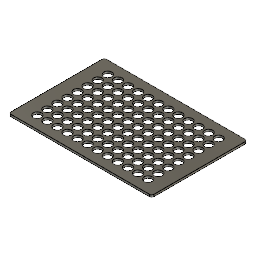
PlateAdaptor_gasket (Autodesk Fusion 360 design; units mm, degrees)
Autodesk Fusion 360 part; units mm, degrees
sketch "Sketch1" plane through (0, 0, 0) normal (0, 0, 1) x (1, 0, 0)
  line L0 (-61.88, 42.735) -> (61.88, 42.735)
  line L1 (63.88, 40.735) -> (63.88, -40.735)
  line L2 (61.88, -42.735) -> (-61.88, -42.735)
  line L3 (-63.88, -40.735) -> (-63.88, 40.735)
  line L4 (-63.88, 42.735) -> (63.88, -42.735) construction
  line L5 (63.88, 42.735) -> (-63.88, -42.735) construction
  line L6 (-48.38, 42.735) -> (-58.38, 42.735)
  line L7 (48.38, -47.37) -> (58.38, -47.37)
  line L8 (-58.38, -47.37) -> (-48.38, -47.37)
  line L9 (-49.5, 31.5) -> (49.5, 31.5)
  line L10 (49.5, 31.5) -> (49.5, -31.5)
  line L11 (49.5, -31.5) -> (-49.5, -31.5)
  line L12 (-49.5, -31.5) -> (-49.5, 31.5)
  line L13 (-49.5, 31.5) -> (49.5, -31.5) construction
  line L14 (49.5, 31.5) -> (-49.5, -31.5) construction
  circle A0 centre (-49.5, -31.5) radius 3.575
  circle A1 centre (-40.5, -31.5) radius 3.575
  circle A2 centre (-31.5, -31.5) radius 3.575
  circle A3 centre (-22.5, -31.5) radius 3.575
  circle A4 centre (-13.5, -31.5) radius 3.575
  circle A5 centre (-4.5, -31.5) radius 3.575
  circle A6 centre (4.5, -31.5) radius 3.575
  circle A7 centre (13.5, -31.5) radius 3.575
  circle A8 centre (22.5, -31.5) radius 3.575
  circle A9 centre (31.5, -31.5) radius 3.575
  circle A10 centre (40.5, -31.5) radius 3.575
  circle A11 centre (49.5, -31.5) radius 3.575
  circle A12 centre (-49.5, -22.5) radius 3.575
  circle A13 centre (-40.5, -22.5) radius 3.575
  circle A14 centre (-31.5, -22.5) radius 3.575
  circle A15 centre (-22.5, -22.5) radius 3.575
  circle A16 centre (-13.5, -22.5) radius 3.575
  circle A17 centre (-4.5, -22.5) radius 3.575
  circle A18 centre (4.5, -22.5) radius 3.575
  circle A19 centre (13.5, -22.5) radius 3.575
  circle A20 centre (22.5, -22.5) radius 3.575
  circle A21 centre (31.5, -22.5) radius 3.575
  circle A22 centre (40.5, -22.5) radius 3.575
  circle A23 centre (49.5, -22.5) radius 3.575
  circle A24 centre (-49.5, -13.5) radius 3.575
  circle A25 centre (-40.5, -13.5) radius 3.575
  circle A26 centre (-31.5, -13.5) radius 3.575
  circle A27 centre (-22.5, -13.5) radius 3.575
  circle A28 centre (-13.5, -13.5) radius 3.575
  circle A29 centre (-4.5, -13.5) radius 3.575
  circle A30 centre (4.5, -13.5) radius 3.575
  circle A31 centre (13.5, -13.5) radius 3.575
  circle A32 centre (22.5, -13.5) radius 3.575
  circle A33 centre (31.5, -13.5) radius 3.575
  circle A34 centre (40.5, -13.5) radius 3.575
  circle A35 centre (49.5, -13.5) radius 3.575
  circle A36 centre (-49.5, -4.5) radius 3.575
  circle A37 centre (-40.5, -4.5) radius 3.575
  circle A38 centre (-31.5, -4.5) radius 3.575
  circle A39 centre (-22.5, -4.5) radius 3.575
  circle A40 centre (-13.5, -4.5) radius 3.575
  circle A41 centre (-4.5, -4.5) radius 3.575
  circle A42 centre (4.5, -4.5) radius 3.575
  circle A43 centre (13.5, -4.5) radius 3.575
  circle A44 centre (22.5, -4.5) radius 3.575
  circle A45 centre (31.5, -4.5) radius 3.575
  circle A46 centre (40.5, -4.5) radius 3.575
  circle A47 centre (49.5, -4.5) radius 3.575
  circle A48 centre (-49.5, 4.5) radius 3.575
  circle A49 centre (-40.5, 4.5) radius 3.575
  circle A50 centre (-31.5, 4.5) radius 3.575
  circle A51 centre (-22.5, 4.5) radius 3.575
  circle A52 centre (-13.5, 4.5) radius 3.575
  circle A53 centre (-4.5, 4.5) radius 3.575
  circle A54 centre (4.5, 4.5) radius 3.575
  circle A55 centre (13.5, 4.5) radius 3.575
  circle A56 centre (22.5, 4.5) radius 3.575
  circle A57 centre (31.5, 4.5) radius 3.575
  circle A58 centre (40.5, 4.5) radius 3.575
  circle A59 centre (49.5, 4.5) radius 3.575
  circle A60 centre (-49.5, 13.5) radius 3.575
  circle A61 centre (-40.5, 13.5) radius 3.575
  circle A62 centre (-31.5, 13.5) radius 3.575
  circle A63 centre (-22.5, 13.5) radius 3.575
  circle A64 centre (-13.5, 13.5) radius 3.575
  circle A65 centre (-4.5, 13.5) radius 3.575
  circle A66 centre (4.5, 13.5) radius 3.575
  circle A67 centre (13.5, 13.5) radius 3.575
  circle A68 centre (22.5, 13.5) radius 3.575
  circle A69 centre (31.5, 13.5) radius 3.575
  circle A70 centre (40.5, 13.5) radius 3.575
  circle A71 centre (49.5, 13.5) radius 3.575
  circle A72 centre (-49.5, 22.5) radius 3.575
  circle A73 centre (-40.5, 22.5) radius 3.575
  circle A74 centre (-31.5, 22.5) radius 3.575
  circle A75 centre (-22.5, 22.5) radius 3.575
  circle A76 centre (-13.5, 22.5) radius 3.575
  circle A77 centre (-4.5, 22.5) radius 3.575
  circle A78 centre (4.5, 22.5) radius 3.575
  circle A79 centre (13.5, 22.5) radius 3.575
  circle A80 centre (22.5, 22.5) radius 3.575
  circle A81 centre (31.5, 22.5) radius 3.575
  circle A82 centre (40.5, 22.5) radius 3.575
  circle A83 centre (49.5, 22.5) radius 3.575
  circle A84 centre (-49.5, 31.5) radius 3.575
  circle A85 centre (-40.5, 31.5) radius 3.575
  circle A86 centre (-31.5, 31.5) radius 3.575
  circle A87 centre (-22.5, 31.5) radius 3.575
  circle A88 centre (-13.5, 31.5) radius 3.575
  circle A89 centre (-4.5, 31.5) radius 3.575
  circle A90 centre (4.5, 31.5) radius 3.575
  circle A91 centre (13.5, 31.5) radius 3.575
  circle A92 centre (22.5, 31.5) radius 3.575
  circle A93 centre (31.5, 31.5) radius 3.575
  circle A94 centre (40.5, 31.5) radius 3.575
  circle A95 centre (49.5, 31.5) radius 3.575
  arc A96 (-61.88, 42.735) -> (-63.88, 40.735) centre (-61.88, 40.735) ccw
  arc A97 (-63.88, -40.735) -> (-61.88, -42.735) centre (-61.88, -40.735) ccw
  arc A98 (61.88, -42.735) -> (63.88, -40.735) centre (61.88, -40.735) ccw
  arc A99 (63.88, 40.735) -> (61.88, 42.735) centre (61.88, 40.735) ccw
  point P0 (-57.3369, -42.2056)
  point P1 (-53.88, -84.89)
  dimension "d1" = 127.76
  dimension "d2" = 85.47
  dimension "d7" = 63
  dimension "d8" = 99
  dimension "d10" = 7.15
  dimension "d13" = 99
  dimension "d14" = 63
  dimension "d15" = 2
  dimension "d16" = 2
  dimension "d17" = 2
  dimension "d18" = 2
  constraint perpendicular L0 L1
  constraint parallel L0 L2
  constraint parallel L1 L3
  constraint horizontal L0
  constraint coincident L4 origin
  constraint coincident L5 origin
  constraint horizontal L6
  constraint coincident L0 L6.start
  constraint horizontal L7
  constraint horizontal L8
  constraint perpendicular L9 L10
  constraint parallel L9 L11
  constraint parallel L10 L12
  constraint horizontal L9
  constraint coincident L13 origin
  constraint coincident L14 origin
  constraint coincident L4.start L0
  constraint coincident L4.start L3
  constraint tangent L0 A96
  constraint tangent L3 A96
  constraint coincident L5.end L3
  constraint coincident L5.end L2
  constraint tangent L3 A97
  constraint tangent L2 A97
  constraint coincident L4.end L2
  constraint coincident L4.end L1
  constraint tangent L2 A98
  constraint tangent L1 A98
  constraint coincident L5.start L0
  constraint coincident L5.start L1
  constraint tangent L0 A99
  constraint tangent L1 A99
  measures "d1" distance of L1 L3
  measures "d2" distance of L4.start L5.end
  measures "d7" distance of L9.end L10.end
  measures "d8" distance of L10.end L11.end
  measures "d10" diameter of A0
  measures "d15" radius of A96
  measures "d16" radius of A97
  measures "d17" radius of A98
  measures "d18" radius of A99
extrude "Extrude1" add sketch "Sketch1" along normal blind 2 contours L0 L1 L2 L3 L6 A96 A97 A98 A99 | L9 L10 L11 L12 A0 A1 A2 A3 A4 A5 A6 A7 A8 A9 A10 A11 A12 A23 A24 A35 A36 A47 A48 A59 A60 A71 A72 A83 A84 A85 A86 A87 A88 A89 A90 A91 A92 A93 A94 A95
